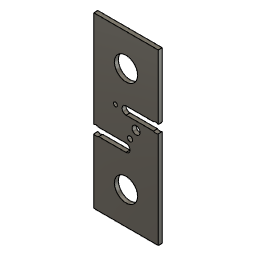
Sandia_2nd_Fracture_Challenge (Autodesk Fusion 360 design; units mm, degrees)
Autodesk Fusion 360 part; units mm, degrees
sketch "Sketch1" plane through (0, 0, 0) normal (0, 0, 1) x (1, 0, 0)
  line L0 (-25.4, 66.675) -> (25.4, 66.675)
  line L1 (25.4, -66.675) -> (-25.4, -66.675)
  circle A0 centre (-8.3186, 12.705) radius 1.59
  circle A1 centre (7.9382, 3.175) radius 3.175
  circle A2 centre (3.17, -5.075) radius 1.995
  arc A3 (-21.5734, -9.515) -> (-25.4, -9.515) centre (-23.4867, -12.055) ccw
  arc A4 (-25.4, -15.875) -> (-21.5734, -15.875) centre (-23.4867, -13.335) ccw
  line L2 (-21.5734, -9.515) -> (0, -9.515)
  arc A5 (0, -15.875) -> (0, -9.515) centre (0, -12.695) ccw
  line L3 (0, -15.875) -> (-21.5734, -15.875)
  line L4 (-25.4, -66.675) -> (-25.4, -15.875)
  line L5 (-25.4, -9.515) -> (-25.4, 66.675)
  arc A6 (25.4, 15.885) -> (21.5734, 15.885) centre (23.4867, 13.345) ccw
  arc A7 (21.5734, 9.525) -> (25.4, 9.525) centre (23.4867, 12.065) ccw
  line L6 (21.5734, 9.525) -> (0, 9.525)
  arc A8 (0, 15.885) -> (0, 9.525) centre (0, 12.705) ccw
  line L7 (0, 15.885) -> (21.5734, 15.885)
  line L8 (25.4, 66.675) -> (25.4, 15.885)
  line L9 (25.4, 9.525) -> (25.4, -66.675)
  line L10 (0, 66.675) -> (0, -66.675) construction
  line L11 (-60, 0) -> (90, 0) construction
  circle A9 centre (0, 41.275) radius 9.145
  circle A10 centre (0, -41.275) radius 9.145
  line L12 (-8.3186, 12.705) -> (0, 12.705) construction
  line L13 (-23.4867, -12.055) -> (-23.4867, -13.335) construction
  line L14 (0, -12.695) -> (-23.4867, -12.695) construction
  line L15 (23.4867, 13.345) -> (23.4867, 12.065) construction
  line L16 (0, 12.705) -> (23.4867, 12.705) construction
  line L17 (-25.4, -9.515) -> (-21.5734, -9.515) construction
  line L18 (21.5734, 15.885) -> (25.4, 15.885) construction
  dimension "d1" = 133.35
  dimension "d2" = 50.8
  dimension "d3" = 3.18
  dimension "d4" = 6.35
  dimension "d5" = 3.99
  dimension "d6" = 3.18
  dimension "d7" = 18.29
  dimension "d8" = 25.4
  dimension "d9" = 25.4
  dimension "d10" = 3.18
  dimension "d11" = 3.18
  dimension "d12" = 53.98
  dimension "d13" = 79.38
  dimension "d14" = 61.6
  dimension "d15" = 69.85
  dimension "d16" = 17.4618
  dimension "d17" = 22.23
  dimension "d18" = 33.7186
  dimension "d19" = 0.64
  dimension "d20" = 0.64
  dimension "d21" = 66.675
  constraint horizontal L0
  constraint vertical L8
  constraint horizontal L1
  constraint vertical L4
  constraint coincident A3.end L4
  constraint horizontal L2
  constraint tangent L2 A5
  constraint horizontal L3
  constraint tangent A5 L3
  constraint collinear L4 L5
  constraint coincident A7.end L8
  constraint horizontal L6
  constraint tangent L6 A8
  constraint horizontal L7
  constraint tangent A8 L7
  constraint collinear L8 L9
  constraint equal A5 A8
  constraint coincident A7.start L6.start
  constraint midpoint L0 L10.start
  constraint midpoint L1 L10.end
  constraint coincident origin L10
  constraint horizontal L11
  constraint coincident origin L11
  constraint coincident L10 A9.centre
  constraint coincident L10 A10.centre
  constraint equal A9 A10
  constraint coincident A5.centre L10
  constraint coincident A8.centre L10
  constraint equal A3 A4
  constraint equal A6 A7
  constraint equal L2 L3
  constraint equal L6 L7
  constraint coincident A0.centre L12.start
  constraint coincident A8.centre L12.end
  constraint horizontal L12
  constraint coincident A3.centre L13.start
  constraint coincident A4.centre L13.end
  constraint vertical L13
  constraint coincident A5.centre L14.start
  constraint midpoint L13 L14.end
  constraint horizontal L14
  constraint coincident A6.centre L15.start
  constraint coincident A7.centre L15.end
  constraint midpoint L15 L16.end
  constraint horizontal L16
  constraint horizontal L17
  constraint horizontal L18
  measures "d1" distance of L0.end L1.start
  measures "d2" distance of L0.start L0.end
  measures "d3" diameter of A0
  measures "d4" diameter of A1
  measures "d5" diameter of A2
  measures "d6" radius of A5
  measures "d7" diameter of A9
  measures "d8" distance of L1 A10.centre
  measures "d9" distance of L0 A9.centre
  measures "d10" radius of A4
  measures "d11" radius of A6
  measures "d12" distance of A5.centre L10.end
  measures "d13" distance of L1 A8.centre
  measures "d14" distance of L1 A2.centre
  measures "d15" distance of L1 A1.centre
  measures "d16" distance of A1.centre L9
  measures "d17" distance of A2.centre L9
  measures "d18" distance of A0.centre L8
  measures "d19" distance of A4.centre L14
  measures "d20" distance of A6.centre L16
  measures "d21" distance of L1 L11
extrude "Extrude1" add sketch "Sketch1" along normal mid plane 3.124
